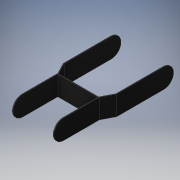
# Autodesk Inventor part: Upper Arm
Saved by Autodesk Inventor 2017 (Build 210142000, 142)
## iProperties
Created: 2018-10-18
Part Number: Upper Arm
Material: Generic
Document SubType Name: Modeling
Designer: Cameron
Density: 1 g/cm^3
Appearance: Glossy - Black
Author: Cameron
Autodesk Inventor part; units mm, degrees
ref_plane "YZ Plane" through (0, 0, 0) normal (1, 0, 0) x (0, 1, 0)
ref_plane "XZ Plane" through (0, 0, 0) normal (0, 1, 0) x (-1, 0, 0)
ref_plane "XY Plane" through (0, 0, 0) normal (0, 0, 1) x (1, 0, 0)
sketch "Sketch1" plane through (0, 0, 0) normal (0, 1, 0) x (-1, 0, 0)
  line L0 (68, 0) -> (68, -145)
  line L1 (68, -145) -> (0, -145)
  line L2 (0, -145) -> (0, 0)
  line L3 (1, -144) -> (67, -144)
  line L4 (60.5, 0) -> (60.5, -58)
  line L5 (59.5, -58) -> (8.5, -58)
  line L6 (7.5, -58) -> (7.5, 0)
  line L7 (8.5, 0) -> (8.5, -57)
  line L8 (8.5, -57) -> (59.5, -57)
  line L9 (59.5, -57) -> (59.5, 0)
  line L10 (7.5, 0) -> (8.5, 0)
  line L11 (59.5, 0) -> (60.5, 0)
  line L12 (7.5, -58) -> (0, -72.5)
  line L13 (8.5, -58) -> (1, -72.5)
  line L14 (60.5, -58) -> (68, -72.5)
  line L15 (67, -72.5) -> (59.5, -58)
  line L16 (67, -145) -> (67, -72.5)
  line L17 (67, -70.5667) -> (67, -1)
  line L18 (1, -1) -> (1, -70.5667)
  line L19 (1, -72.5) -> (1, -145)
  dimension "d0" = 68
  dimension "d1" = 145
  dimension "d4" = 58
  dimension "d5" = 53
  dimension "d6" = 1
  constraints: 40 end point, 8 parallel, 6 perpendicular, 6 point on line, 2 horizontal, 2 midpoint
  measures "d0" distance of L0.end L1.end
  measures "d1" distance of L0.start L0.end
  measures "d4" distance of L4.start L4.end
  measures "d5" distance of L4.end L6.start
  measures "d6" distance between parallel lines of L6 L7
extrude "Extrusion1" add sketch "Sketch1" along normal blind 25 contours L0 L1 L16 L15 L5 L13 L19 L2 L12 L6 L10 L7 L8 L9 L11 L4 L14
fillet "Fillet1" radius 12.5 8 edges at (-8, 25, 0) (-8, 0, 0) (-60, 0, 0) (-60, 25, 0) (-0.5, 25, -145) (-67.5, 25, -145) (-67.5, 0, -145) (-0.5, 0, -145)
body "Solid1"
